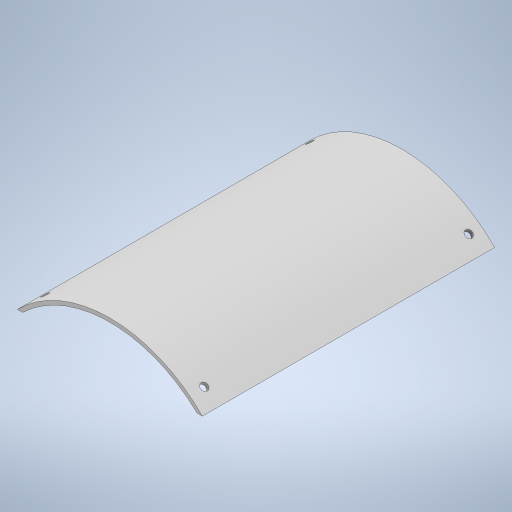
# Autodesk Inventor part: Electronics Door
Saved by Autodesk Inventor 2024 (Build 280153000, 153)
## iProperties
Created: 2024-04-23
Part Number: Electronics Door
Material: Generic
Document SubType Name: Modeling
Designer: auror
Density: 1 g/cm^3
Appearance: Default
Author: auror
Autodesk Inventor part; units mm, degrees
ref_plane "YZ Plane" through (0, 0, 0) normal (1, 0, 0) x (0, 1, 0)
sketch "Sketch8" plane through (0, 0, 0) normal (0, 0, 1) x (1, 0, 0)
  arc A0 (23.5572, 24.5165) -> (-23.5572, 24.5165) centre (0, 0) ccw
  arc A1 (25, 24.4949) -> (-25, 24.4949) centre (0, 0) ccw
  line L0 (-23.5572, 24.5165) -> (-25, 24.4949)
  line L1 (-24.431, 23.6769) -> (-22.7081, 25.3323) construction
  line L2 (22.7844, 25.2591) -> (24.3419, 23.7625) construction
  line L3 (23.5572, 24.5165) -> (25, 24.4949)
  line L4 (-25, 24.4949) -> (25, 24.4949) construction
  dimension "d88" = 34
  dimension "d89" = 35
  dimension "d90" = 0
  dimension "d91" = 137
  dimension "d92" = 0
  dimension "d93" = 137
  dimension "d98" = 50
  constraints: 10 end point, 4 point on circle, 2 centre point, 2 coincident, 2 tangent, 1 horizontal
  measures "d88" radius of A0
  measures "d89" radius of A1
  measures "d90" distance from line of L0.start L1
  measures "d91" angle of L0 L1
  measures "d92" distance from line of L3.start L2
  measures "d93" angle of L3 L2
  measures "d98" distance of L0.end L3.end
extrude "Extrusion5" add sketch "Sketch8" along normal blind 79
sketch "Sketch19" plane through (0, 0, 79) normal (0, 0, 1) x (1, 0, 0)
  line L0 (-25, 24.4949) -> (-23.5572, 24.5165) construction
  line L1 (-22.2755, 25.021) -> (-7.4699, 32.6566) construction
  arc A0 (22.2755, 25.021) -> (-22.2755, 25.021) centre (0, 0) ccw construction
  dimension "d162" = 32.448
  constraints: 2 end point, 1 point on circle, 1 other
  measures "d162" distance from line of point (0, 0) L1
sketch "Sketch22" plane through (0, 0, 79) normal (0, 0, 1) x (1, 0, 0)
  line L0 (0, 0) -> (23.9071, 24.8806) construction
  line L1 (0, 0) -> (31.302, 21.2274) construction
  arc A0 (23.5572, 24.5165) -> (-23.5572, 24.5165) centre (0, 0) ccw construction
  arc A1 (29.7973, 16.3744) -> (23.5572, 24.5165) centre (0, 0) ccw construction
  line L2 (28.1397, 19.0829) -> (9.553, 32.6304) construction
  point P0 (19.5664, 25.3318)
  dimension "d175" = 12
  dimension "d176" = 23
  dimension "d177" = 0
  dimension "d178" = 10.609
  constraints: 6 end point, 4 point on circle, 2 point on line, 1 centre point, 1 coincident
  measures "d175" angle of L0 L1
  measures "d176" distance of L2.start L2.end
  measures "d177" distance from line of A0.start L0
  measures "d178" distance of L2.start point (19.566, 25.332)
sketch "Sketch23" plane through (0, 0, 0) normal (0, 0, -1) x (-1, 0, 0)
  arc A0 (23.5572, 24.5165) -> (-23.5572, 24.5165) centre (0, 0) ccw projected
  line L0 (0, 0) -> (-23.5572, 24.5165) construction
  line L1 (0, 0) -> (-31.0154, 21.0331) construction
  arc A1 (-23.5572, 24.5165) -> (-29.6271, 16.6805) centre (0, 0) ccw construction
  line L2 (-28.1397, 19.0829) -> (-9.553, 32.6304) construction
  dimension "d179" = 12
  dimension "d180" = 23
  constraints: 6 end point, 4 point on circle, 1 centre point, 1 coincident, 1 point on line
  measures "d179" angle of L0 L1
  measures "d180" distance of L2.start L2.end
ref_plane "Work Plane12" through (28.1397, 19.0829, 79) normal (-0.589, -0.8081, 0) x (-0.8081, 0.589, 0)
sketch "Sketch24" plane through (28.1397, 19.0829, 79) normal (-0.589, -0.8081, 0) x (-0.8081, 0.589, 0)
  line L0 (6.9037, 79) -> (6.9037, 0) projected
  line L1 (44.9777, 0) -> (6.9037, 0) projected
  line L2 (44.9777, 79) -> (6.9037, 79) projected
  point P0 (11.5, 79)
  point P1 (10.4037, 75.5)
  point P2 (10.4037, 4)
  dimension "d181" = 3.5
  dimension "d182" = 4
  dimension "d183" = 3.5
  dimension "d184" = 3.5
  measures "d181" distance from line of L0 point (10.404, 4)
  measures "d182" distance from line of point (10.404, 4) L1
  measures "d183" distance from line of L2 point (10.404, 75.5)
  measures "d184" distance from line of L0 point (10.404, 75.5)
hole "Hole11" at (19.7323, 25.2109, 3.5) at (19.7323, 25.2109, 75) direction (0.589, 0.8081, 0) diameter 2 end through all
ref_plane "Work Plane13" through (0, 24.8688, 0) normal (1, 0, 0) x (0, 0, 1)
mirror "Mirror2" about plane through (0, 24.8688, 0) normal (1, 0, 0) of "Hole11"
body "Solid2"
